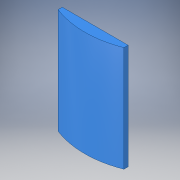
# Autodesk Inventor part: 00_Comar_Lens_Cylindrical_50mm
Saved by Autodesk Inventor 2019 (Build 230136000, 136)
## iProperties
Created: 2019-08-29
Part Number: 00_Comar_Lens_Cylindrical_50mm
Material: Glass
Document SubType Name: Modeling
Designer: diederichbenedict
Density: 2.18 g/cm^3
Appearance: Cyan
Author: diederichbenedict
Autodesk Inventor part; units mm, degrees
ref_plane "YZ Plane" through (0, 0, 0) normal (1, 0, 0) x (0, 1, 0)
ref_plane "XZ Plane" through (0, 0, 0) normal (0, 1, 0) x (-1, 0, 0)
ref_plane "XY Plane" through (0, 0, 0) normal (0, 0, 1) x (1, 0, 0)
sketch "Sketch1" plane through (0, 0, 0) normal (0, 1, 0) x (-1, 0, 0)
  line L0 (0, 0) -> (25, 0)
  line L1 (25, 0) -> (25, 1.59)
  line L2 (25, 1.59) -> (0, 1.59)
  line L3 (0, 1.59) -> (0, 0)
  arc A0 (25, 1.59) -> (0, 1.59) centre (12.5, -30.3338) ccw
  line L4 (12.5, 0) -> (12.5, 3.95) construction
  dimension "d0" = 25
  dimension "d1" = 1.59
  dimension "d6" = 3.95
  constraints: 10 end point, 3 point on circle, 2 parallel, 1 centre point, 1 horizontal, 1 midpoint, 1 perpendicular
  measures "d0" distance of L2.end L1.end
  measures "d1" distance of L1.end L0.end
  measures "d6" distance of L4.start L4.end
extrude "Extrusion1" add sketch "Sketch1" along normal blind 40
sketch "Sketch2" plane through (0, 0, 0) normal (0, 0, -1) x (-1, 0, 0)
  line L0 (0, 0) -> (25, 0) projected
  line L1 (25, 0) -> (25, 40) projected
  line L2 (0, 40) -> (25, 40) projected
  line L3 (0, 0) -> (0, 40) projected
  circle A0 centre (12.5, 20) radius 1.6121
  constraints: 1 centre point
extrude "Extrusion2" [suppressed]
sketch "Sketch3" plane through (0, 0, 0) normal (0, 0, -1) x (-1, 0, 0)
  line L0 (0, 0) -> (25, 0) construction
  line L1 (25, 0) -> (25, 40) construction
  line L2 (0, 40) -> (25, 40) construction
  line L3 (0, 0) -> (0, 40) construction
  line L4 (0, 40) -> (25, 0) construction
  line L5 (25, 0) -> (25, 40) construction
  line L6 (25, 40) -> (0, 0) construction
  point P0 (12.5, 20)
  constraints: 4 end point, 2 midpoint
body "Solid1"
